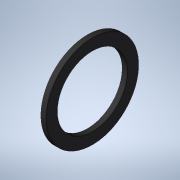
# Autodesk Inventor part: GS81110Outer Rings
Saved by Autodesk Inventor 2021 (Build 250183000, 183)
## iProperties
Created: 2025-09-20
Part Number: GS81110Outer Rings
Material: Generic
Catalog Web Link: www.cadenas.de
Description: GS811,GS812,GS893 (Outer rings)-
Vendor: NTN
Document SubType Name: Modeling
Designer: psAdmin
Manufacturer: NTN
Mass: 6.86933 g
Surface Area: 48.8386 cm^2
Volume: 6.86933 cm^3
Density: 1 g/cm^3
Appearance: PSOLRGB-175-175-175
Category: PARTsolutions
Company: NTN
Title: GS81110
Author: Cadenas PARTsolutions
PSOL_IDENT_0: {$CADENAS_DATA/23d-libs/ntn/needle_roler_bearings/cylindrical_roler_thrust_b/gs811_gs812_gs893_or.pr
PSOL_IDENT_1: j},191 {VTYP=3D},{NB=GS81110Outer Rings},{LINA=GS81110},{NN=GS811,GS812,GS893 (Outer rings)},{DATE=2
PSOL_IDENT_2: 3.07.2025 07:07:17},{GEOMDATE=20.04.2020 04:44:19},{VERSION=},{LINEID=190},{WBVAR=},{WBNUMERIC=}  {N
PSOL_IDENT_3: B=GS81110Outer Rings},{LINA=GS81110},{KT=DUMMY},{ORDER=GS81110},{D1=52},{D=70},{B=4.00},{R=0.6},{CA=
PSOL_IDENT_4: 48500},{COA=150000},{CAF=4900},{COAF=15300},{LSG=1000},{LSO=4000},{MASS=0.054}
NB: GS81110Outer Rings
NN: GS811,GS812,GS893 (Outer rings)
NBSYN: $ORDER.Outer Rings
LINA: GS81110
CATALOG: NTN Corporation
ORDER: GS81110
D1: 52
D: 70
B: 4
R: 0.6
MASS: 0.054
SUPPLIER: NTN
ARTICLENO: GS81110Outer Rings
BOMINFO: GS81110
CREATOR: CADENAS GmbH
Autodesk Inventor part; units mm, degrees
ref_plane "YZ Plane" through (0, 0, 0) normal (1, 0, 0) x (0, 1, 0)
ref_plane "XZ Plane" through (0, 0, 0) normal (0, 1, 0) x (-1, 0, 0)
ref_plane "XY Plane" through (0, 0, 0) normal (0, 0, 1) x (1, 0, 0)
sketch "Sketch_1" plane through (0, 0, 0) normal (0, 0, 1) x (1, 0, 0)
  line L0 (4, 0) -> (0, 0)
  line L1 (0, 26) -> (3.4, 26)
  arc A0 (3.4, 26) -> (4, 26.6) centre (3.4, 26.6) ccw
  line L2 (4, 26.6) -> (4, 34.4)
  arc A1 (4, 34.4) -> (3.4, 35) centre (3.4, 34.4) ccw
  line L3 (3.4, 35) -> (0, 35)
  line L4 (0, 35) -> (0, 26)
  constraints: 10 end point, 4 point on circle, 2 centre point
revolve "Revolution1" add sketch "Sketch_1" angle 360 about axis through (4, 0, 0) along (1, 0, 0)
body "Solid1"
